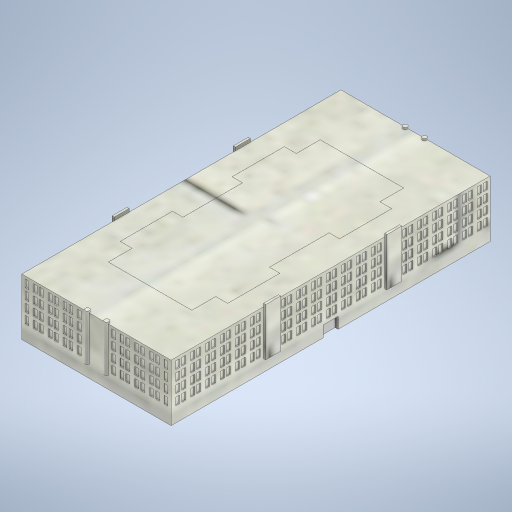
# Autodesk Inventor part: 底部
Saved by Autodesk Inventor 2024.2 (Build 282272000, 272)
## iProperties
Created: 2024-05-15
Part Number: 底部
Material: 一般
Document SubType Name: Modeling
Designer: sohil
Density: 1 g/cm^3
Appearance: 預設
Author: sohil
Autodesk Inventor part; units mm, degrees
(part 1 of 2)
ref_plane "YZ Plane" through (0, 0, 0) normal (1, 0, 0) x (0, 1, 0)
sketch "草圖1" plane through (0, 0, 0) normal (0, 1, 0) x (-1, 0, 0)
  line L0 (20.1844, 27.5664) -> (-79.8156, 27.5664)
  line L1 (-79.8156, 27.5664) -> (-79.8156, -186.2336)
  line L2 (-79.8156, -186.2336) -> (20.1844, -186.2336)
  line L3 (20.1844, -186.2336) -> (20.1844, 27.5664)
  point P0 (0, 0)
  dimension "d0" = 100
  dimension "d1" = 213.8
  constraints: 8 end point, 2 parallel, 1 horizontal, 1 perpendicular
  measures "d0" distance of L2.end L1.end
  measures "d1" distance of L1.end L0.end
extrude "擠出1" add sketch "草圖1" along normal blind 30
sketch "草圖5" plane through (-20.1844, 0, -186.2336) normal (-1, 0, 0) x (0, 0, 1)
  line L0 (1.8826, 27.9757) -> (4.3826, 27.9757)
  line L1 (4.3826, 27.9757) -> (4.3826, 22.9757)
  line L2 (4.3826, 22.9757) -> (1.8826, 22.9757)
  line L3 (1.8826, 22.9757) -> (1.8826, 27.9757)
  line L4 (5.8826, 27.9757) -> (8.3826, 27.9757)
  line L5 (8.3826, 27.9757) -> (8.3826, 22.9757)
  line L6 (8.3826, 22.9757) -> (5.8826, 22.9757)
  line L7 (5.8826, 22.9757) -> (5.8826, 27.9757)
  line L8 (1.8826, 20.9757) -> (4.3826, 20.9757)
  line L9 (4.3826, 20.9757) -> (4.3826, 15.9757)
  line L10 (4.3826, 15.9757) -> (1.8826, 15.9757)
  line L11 (1.8826, 15.9757) -> (1.8826, 20.9757)
  line L12 (5.8826, 20.9757) -> (8.3826, 20.9757)
  line L13 (8.3826, 20.9757) -> (8.3826, 15.9757)
  line L14 (8.3826, 15.9757) -> (5.8826, 15.9757)
  line L15 (5.8826, 15.9757) -> (5.8826, 20.9757)
  line L16 (1.8826, 13.9757) -> (4.3826, 13.9757)
  line L17 (4.3826, 13.9757) -> (4.3826, 8.9757)
  line L18 (4.3826, 8.9757) -> (1.8826, 8.9757)
  line L19 (1.8826, 8.9757) -> (1.8826, 13.9757)
  line L20 (5.8826, 13.9757) -> (8.3826, 13.9757)
  line L21 (8.3826, 13.9757) -> (8.3826, 8.9757)
  line L22 (8.3826, 8.9757) -> (5.8826, 8.9757)
  line L23 (5.8826, 8.9757) -> (5.8826, 13.9757)
  line L24 (1.8826, 6.9757) -> (4.3826, 6.9757)
  line L25 (4.3826, 6.9757) -> (4.3826, 1.9757)
  line L26 (4.3826, 1.9757) -> (1.8826, 1.9757)
  line L27 (1.8826, 1.9757) -> (1.8826, 6.9757)
  line L28 (5.8826, 6.9757) -> (8.3826, 6.9757)
  line L29 (8.3826, 6.9757) -> (8.3826, 1.9757)
  line L30 (8.3826, 1.9757) -> (5.8826, 1.9757)
  line L31 (5.8826, 1.9757) -> (5.8826, 6.9757)
  line L32 (11.8826, 27.9757) -> (14.3826, 27.9757)
  line L33 (11.8826, 22.9757) -> (11.8826, 27.9757)
  line L34 (14.3826, 27.9757) -> (14.3826, 22.9757)
  line L35 (15.8826, 27.9757) -> (18.3826, 27.9757)
  line L36 (15.8826, 22.9757) -> (15.8826, 27.9757)
  line L37 (18.3826, 27.9757) -> (18.3826, 22.9757)
  line L38 (18.3826, 22.9757) -> (15.8826, 22.9757)
  line L39 (14.3826, 22.9757) -> (11.8826, 22.9757)
  line L40 (11.8826, 20.9757) -> (14.3826, 20.9757)
  line L41 (11.8826, 15.9757) -> (11.8826, 20.9757)
  line L42 (14.3826, 20.9757) -> (14.3826, 15.9757)
  line L43 (14.3826, 15.9757) -> (11.8826, 15.9757)
  line L44 (15.8826, 15.9757) -> (15.8826, 20.9757)
  line L45 (15.8826, 20.9757) -> (18.3826, 20.9757)
  line L46 (18.3826, 20.9757) -> (18.3826, 15.9757)
  line L47 (18.3826, 15.9757) -> (15.8826, 15.9757)
  line L48 (11.8826, 13.9757) -> (14.3826, 13.9757)
  line L49 (11.8826, 8.9757) -> (11.8826, 13.9757)
  line L50 (14.3826, 8.9757) -> (11.8826, 8.9757)
  line L51 (14.3826, 13.9757) -> (14.3826, 8.9757)
  line L52 (11.8826, 1.9757) -> (11.8826, 6.9757)
  line L53 (14.3826, 1.9757) -> (11.8826, 1.9757)
  line L54 (14.3826, 6.9757) -> (14.3826, 1.9757)
  line L55 (11.8826, 6.9757) -> (14.3826, 6.9757)
  line L56 (18.3826, 6.9757) -> (18.3826, 1.9757)
  line L57 (15.8826, 6.9757) -> (18.3826, 6.9757)
  line L58 (15.8826, 1.9757) -> (15.8826, 6.9757)
  line L59 (18.3826, 1.9757) -> (15.8826, 1.9757)
  line L60 (15.8826, 8.9757) -> (15.8826, 13.9757)
  line L61 (18.3826, 8.9757) -> (15.8826, 8.9757)
  line L62 (18.3826, 13.9757) -> (18.3826, 8.9757)
  line L63 (15.8826, 13.9757) -> (18.3826, 13.9757)
  line L64 (21.8826, 27.9757) -> (24.3826, 27.9757)
  line L65 (21.8826, 22.9757) -> (21.8826, 27.9757)
  line L66 (24.3826, 27.9757) -> (24.3826, 22.9757)
  line L67 (25.8826, 27.9757) -> (28.3826, 27.9757)
  line L68 (25.8826, 22.9757) -> (25.8826, 27.9757)
  line L69 (28.3826, 27.9757) -> (28.3826, 22.9757)
  line L70 (28.3826, 22.9757) -> (25.8826, 22.9757)
  line L71 (24.3826, 22.9757) -> (21.8826, 22.9757)
  line L72 (21.8826, 20.9757) -> (24.3826, 20.9757)
  line L73 (21.8826, 15.9757) -> (21.8826, 20.9757)
  line L74 (24.3826, 20.9757) -> (24.3826, 15.9757)
  line L75 (24.3826, 15.9757) -> (21.8826, 15.9757)
  line L76 (25.8826, 15.9757) -> (25.8826, 20.9757)
  line L77 (25.8826, 20.9757) -> (28.3826, 20.9757)
  line L78 (28.3826, 20.9757) -> (28.3826, 15.9757)
  line L79 (28.3826, 15.9757) -> (25.8826, 15.9757)
  line L80 (21.8826, 13.9757) -> (24.3826, 13.9757)
  line L81 (21.8826, 8.9757) -> (21.8826, 13.9757)
  line L82 (24.3826, 8.9757) -> (21.8826, 8.9757)
  line L83 (24.3826, 13.9757) -> (24.3826, 8.9757)
  line L84 (21.8826, 1.9757) -> (21.8826, 6.9757)
  line L85 (24.3826, 1.9757) -> (21.8826, 1.9757)
  line L86 (24.3826, 6.9757) -> (24.3826, 1.9757)
  line L87 (21.8826, 6.9757) -> (24.3826, 6.9757)
  line L88 (28.3826, 6.9757) -> (28.3826, 1.9757)
  line L89 (25.8826, 6.9757) -> (28.3826, 6.9757)
  line L90 (25.8826, 1.9757) -> (25.8826, 6.9757)
  line L91 (28.3826, 1.9757) -> (25.8826, 1.9757)
  line L92 (25.8826, 8.9757) -> (25.8826, 13.9757)
  line L93 (28.3826, 8.9757) -> (25.8826, 8.9757)
  line L94 (28.3826, 13.9757) -> (28.3826, 8.9757)
  line L95 (25.8826, 13.9757) -> (28.3826, 13.9757)
  line L96 (31.8826, 27.9757) -> (34.3826, 27.9757)
  line L97 (31.8826, 22.9757) -> (31.8826, 27.9757)
  line L98 (34.3826, 27.9757) -> (34.3826, 22.9757)
  line L99 (35.8826, 27.9757) -> (38.3826, 27.9757)
  line L100 (35.8826, 22.9757) -> (35.8826, 27.9757)
  line L101 (38.3826, 27.9757) -> (38.3826, 22.9757)
  line L102 (38.3826, 22.9757) -> (35.8826, 22.9757)
  line L103 (34.3826, 22.9757) -> (31.8826, 22.9757)
  line L104 (31.8826, 20.9757) -> (34.3826, 20.9757)
  line L105 (31.8826, 15.9757) -> (31.8826, 20.9757)
  line L106 (34.3826, 20.9757) -> (34.3826, 15.9757)
  line L107 (34.3826, 15.9757) -> (31.8826, 15.9757)
  line L108 (35.8826, 15.9757) -> (35.8826, 20.9757)
  line L109 (35.8826, 20.9757) -> (38.3826, 20.9757)
  line L110 (38.3826, 20.9757) -> (38.3826, 15.9757)
  line L111 (38.3826, 15.9757) -> (35.8826, 15.9757)
  line L112 (31.8826, 13.9757) -> (34.3826, 13.9757)
  line L113 (31.8826, 8.9757) -> (31.8826, 13.9757)
  line L114 (34.3826, 8.9757) -> (31.8826, 8.9757)
  line L115 (34.3826, 13.9757) -> (34.3826, 8.9757)
  line L116 (31.8826, 1.9757) -> (31.8826, 6.9757)
  line L117 (34.3826, 1.9757) -> (31.8826, 1.9757)
  line L118 (34.3826, 6.9757) -> (34.3826, 1.9757)
  line L119 (31.8826, 6.9757) -> (34.3826, 6.9757)
  line L120 (38.3826, 6.9757) -> (38.3826, 1.9757)
  line L121 (35.8826, 6.9757) -> (38.3826, 6.9757)
  line L122 (35.8826, 1.9757) -> (35.8826, 6.9757)
  line L123 (38.3826, 1.9757) -> (35.8826, 1.9757)
  line L124 (35.8826, 8.9757) -> (35.8826, 13.9757)
  line L125 (38.3826, 8.9757) -> (35.8826, 8.9757)
  line L126 (38.3826, 13.9757) -> (38.3826, 8.9757)
  line L127 (35.8826, 13.9757) -> (38.3826, 13.9757)
  line L128 (41.8826, 27.9757) -> (44.3826, 27.9757)
  line L129 (41.8826, 22.9757) -> (41.8826, 27.9757)
  line L130 (44.3826, 27.9757) -> (44.3826, 22.9757)
  line L131 (45.8826, 27.9757) -> (48.3826, 27.9757)
  line L132 (45.8826, 22.9757) -> (45.8826, 27.9757)
  line L133 (48.3826, 27.9757) -> (48.3826, 22.9757)
  line L134 (48.3826, 22.9757) -> (45.8826, 22.9757)
  line L135 (44.3826, 22.9757) -> (41.8826, 22.9757)
  line L136 (41.8826, 20.9757) -> (44.3826, 20.9757)
  line L137 (41.8826, 15.9757) -> (41.8826, 20.9757)
  line L138 (44.3826, 20.9757) -> (44.3826, 15.9757)
  line L139 (44.3826, 15.9757) -> (41.8826, 15.9757)
  line L140 (45.8826, 15.9757) -> (45.8826, 20.9757)
  line L141 (45.8826, 20.9757) -> (48.3826, 20.9757)
  line L142 (48.3826, 20.9757) -> (48.3826, 15.9757)
  line L143 (48.3826, 15.9757) -> (45.8826, 15.9757)
  line L144 (41.8826, 13.9757) -> (44.3826, 13.9757)
  line L145 (41.8826, 8.9757) -> (41.8826, 13.9757)
  line L146 (44.3826, 8.9757) -> (41.8826, 8.9757)
  line L147 (44.3826, 13.9757) -> (44.3826, 8.9757)
  line L148 (41.8826, 1.9757) -> (41.8826, 6.9757)
  line L149 (44.3826, 1.9757) -> (41.8826, 1.9757)
  line L150 (44.3826, 6.9757) -> (44.3826, 1.9757)
  line L151 (41.8826, 6.9757) -> (44.3826, 6.9757)
  line L152 (48.3826, 6.9757) -> (48.3826, 1.9757)
  line L153 (45.8826, 6.9757) -> (48.3826, 6.9757)
  line L154 (45.8826, 1.9757) -> (45.8826, 6.9757)
  line L155 (48.3826, 1.9757) -> (45.8826, 1.9757)
  line L156 (45.8826, 8.9757) -> (45.8826, 13.9757)
  line L157 (48.3826, 8.9757) -> (45.8826, 8.9757)
  line L158 (48.3826, 13.9757) -> (48.3826, 8.9757)
  line L159 (45.8826, 13.9757) -> (48.3826, 13.9757)
  line L160 (51.8826, 27.9757) -> (54.3826, 27.9757)
  line L161 (51.8826, 22.9757) -> (51.8826, 27.9757)
  line L162 (54.3826, 27.9757) -> (54.3826, 22.9757)
  line L163 (55.8826, 27.9757) -> (58.3826, 27.9757)
  line L164 (55.8826, 22.9757) -> (55.8826, 27.9757)
  line L165 (58.3826, 27.9757) -> (58.3826, 22.9757)
  line L166 (58.3826, 22.9757) -> (55.8826, 22.9757)
  line L167 (54.3826, 22.9757) -> (51.8826, 22.9757)
  line L168 (51.8826, 20.9757) -> (54.3826, 20.9757)
  line L169 (51.8826, 15.9757) -> (51.8826, 20.9757)
  line L170 (54.3826, 20.9757) -> (54.3826, 15.9757)
  line L171 (54.3826, 15.9757) -> (51.8826, 15.9757)
  line L172 (55.8826, 15.9757) -> (55.8826, 20.9757)
  line L173 (55.8826, 20.9757) -> (58.3826, 20.9757)
  line L174 (58.3826, 20.9757) -> (58.3826, 15.9757)
  line L175 (58.3826, 15.9757) -> (55.8826, 15.9757)
  line L176 (51.8826, 13.9757) -> (54.3826, 13.9757)
  line L177 (51.8826, 8.9757) -> (51.8826, 13.9757)
  line L178 (54.3826, 8.9757) -> (51.8826, 8.9757)
  line L179 (54.3826, 13.9757) -> (54.3826, 8.9757)
  line L180 (51.8826, 1.9757) -> (51.8826, 6.9757)
  line L181 (54.3826, 1.9757) -> (51.8826, 1.9757)
  line L182 (54.3826, 6.9757) -> (54.3826, 1.9757)
  line L183 (51.8826, 6.9757) -> (54.3826, 6.9757)
  line L184 (58.3826, 6.9757) -> (58.3826, 1.9757)
  line L185 (55.8826, 6.9757) -> (58.3826, 6.9757)
  line L186 (55.8826, 1.9757) -> (55.8826, 6.9757)
  line L187 (58.3826, 1.9757) -> (55.8826, 1.9757)
  line L188 (55.8826, 8.9757) -> (55.8826, 13.9757)
  line L189 (58.3826, 8.9757) -> (55.8826, 8.9757)
  line L190 (58.3826, 13.9757) -> (58.3826, 8.9757)
  line L191 (55.8826, 13.9757) -> (58.3826, 13.9757)
  line L192 (213.8, 0) -> (0, 0) projected
  line L193 (60.6612, 32.0439) -> (70.6612, 32.0439)
  line L194 (70.6612, 32.0439) -> (70.6612, 0)
  line L195 (70.6612, 0) -> (60.6612, 0)
  line L196 (60.6612, 0) -> (60.6612, 32.0439)
  line L197 (73.0512, 27.9757) -> (75.5512, 27.9757)
  line L198 (75.5512, 27.9757) -> (75.5512, 22.9757)
  line L199 (75.5512, 22.9757) -> (73.0512, 22.9757)
  line L200 (73.0512, 22.9757) -> (73.0512, 27.9757)
  line L201 (77.0512, 27.9757) -> (79.5512, 27.9757)
  line L202 (77.0512, 22.9757) -> (77.0512, 27.9757)
  line L203 (79.5512, 27.9757) -> (79.5512, 22.9757)
  line L204 (79.5512, 22.9757) -> (77.0512, 22.9757)
  line L205 (73.0512, 20.9757) -> (75.5512, 20.9757)
  line L206 (73.0512, 15.9757) -> (73.0512, 20.9757)
  line L207 (75.5512, 20.9757) -> (75.5512, 15.9757)
  line L208 (75.5512, 15.9757) -> (73.0512, 15.9757)
  line L209 (77.0512, 20.9757) -> (79.5512, 20.9757)
  line L210 (77.0512, 15.9757) -> (77.0512, 20.9757)
  line L211 (79.5512, 20.9757) -> (79.5512, 15.9757)
  line L212 (79.5512, 15.9757) -> (77.0512, 15.9757)
  line L213 (73.0512, 13.9757) -> (75.5512, 13.9757)
  line L214 (73.0512, 8.9757) -> (73.0512, 13.9757)
  line L215 (75.5512, 13.9757) -> (75.5512, 8.9757)
  line L216 (75.5512, 8.9757) -> (73.0512, 8.9757)
  line L217 (77.0512, 13.9757) -> (79.5512, 13.9757)
  line L218 (77.0512, 8.9757) -> (77.0512, 13.9757)
  line L219 (79.5512, 13.9757) -> (79.5512, 8.9757)
  line L220 (79.5512, 8.9757) -> (77.0512, 8.9757)
  line L221 (73.0512, 6.9757) -> (75.5512, 6.9757)
  line L222 (73.0512, 1.9757) -> (73.0512, 6.9757)
  line L223 (75.5512, 6.9757) -> (75.5512, 1.9757)
  line L224 (75.5512, 1.9757) -> (73.0512, 1.9757)
  line L225 (77.0512, 6.9757) -> (79.5512, 6.9757)
  line L226 (77.0512, 1.9757) -> (77.0512, 6.9757)
  line L227 (79.5512, 6.9757) -> (79.5512, 1.9757)
  line L228 (79.5512, 1.9757) -> (77.0512, 1.9757)
  line L229 (89.5512, 22.9757) -> (87.0512, 22.9757)
  line L230 (85.5512, 22.9757) -> (83.0512, 22.9757)
  line L231 (83.0512, 22.9757) -> (83.0512, 27.9757)
  line L232 (83.0512, 27.9757) -> (85.5512, 27.9757)
  line L233 (85.5512, 27.9757) -> (85.5512, 22.9757)
  line L234 (87.0512, 27.9757) -> (89.5512, 27.9757)
  line L235 (89.5512, 27.9757) -> (89.5512, 22.9757)
  line L236 (87.0512, 22.9757) -> (87.0512, 27.9757)
  line L237 (83.0512, 13.9757) -> (85.5512, 13.9757)
  line L238 (87.0512, 13.9757) -> (89.5512, 13.9757)
  line L239 (89.5512, 8.9757) -> (87.0512, 8.9757)
  line L240 (89.5512, 13.9757) -> (89.5512, 8.9757)
  line L241 (87.0512, 8.9757) -> (87.0512, 13.9757)
  line L242 (85.5512, 13.9757) -> (85.5512, 8.9757)
  line L243 (85.5512, 8.9757) -> (83.0512, 8.9757)
  line L244 (83.0512, 8.9757) -> (83.0512, 13.9757)
  line L245 (83.0512, 6.9757) -> (85.5512, 6.9757)
  line L246 (87.0512, 6.9757) -> (89.5512, 6.9757)
  line L247 (89.5512, 6.9757) -> (89.5512, 1.9757)
  line L248 (89.5512, 1.9757) -> (87.0512, 1.9757)
  line L249 (83.0512, 1.9757) -> (83.0512, 6.9757)
  line L250 (85.5512, 6.9757) -> (85.5512, 1.9757)
  line L251 (87.0512, 1.9757) -> (87.0512, 6.9757)
  line L252 (85.5512, 1.9757) -> (83.0512, 1.9757)
  line L253 (83.0512, 20.9757) -> (85.5512, 20.9757)
  line L254 (87.0512, 20.9757) -> (89.5512, 20.9757)
  line L255 (89.5512, 15.9757) -> (87.0512, 15.9757)
  line L256 (89.5512, 20.9757) -> (89.5512, 15.9757)
  line L257 (87.0512, 15.9757) -> (87.0512, 20.9757)
  line L258 (85.5512, 20.9757) -> (85.5512, 15.9757)
  line L259 (83.0512, 15.9757) -> (83.0512, 20.9757)
  line L260 (85.5512, 15.9757) -> (83.0512, 15.9757)
  line L261 (99.5512, 22.9757) -> (97.0512, 22.9757)
  line L262 (95.5512, 22.9757) -> (93.0512, 22.9757)
  line L263 (93.0512, 22.9757) -> (93.0512, 27.9757)
  line L264 (93.0512, 27.9757) -> (95.5512, 27.9757)
  line L265 (95.5512, 27.9757) -> (95.5512, 22.9757)
  line L266 (97.0512, 27.9757) -> (99.5512, 27.9757)
  line L267 (99.5512, 27.9757) -> (99.5512, 22.9757)
  line L268 (97.0512, 22.9757) -> (97.0512, 27.9757)
  line L269 (93.0512, 13.9757) -> (95.5512, 13.9757)
  line L270 (97.0512, 13.9757) -> (99.5512, 13.9757)
  line L271 (99.5512, 8.9757) -> (97.0512, 8.9757)
  line L272 (99.5512, 13.9757) -> (99.5512, 8.9757)
  line L273 (97.0512, 8.9757) -> (97.0512, 13.9757)
  line L274 (95.5512, 13.9757) -> (95.5512, 8.9757)
  line L275 (95.5512, 8.9757) -> (93.0512, 8.9757)
  line L276 (93.0512, 8.9757) -> (93.0512, 13.9757)
  line L277 (93.0512, 6.9757) -> (95.5512, 6.9757)
  line L278 (97.0512, 6.9757) -> (99.5512, 6.9757)
  line L279 (99.5512, 6.9757) -> (99.5512, 1.9757)
  line L280 (99.5512, 1.9757) -> (97.0512, 1.9757)
  line L281 (93.0512, 1.9757) -> (93.0512, 6.9757)
  line L282 (95.5512, 6.9757) -> (95.5512, 1.9757)
  line L283 (97.0512, 1.9757) -> (97.0512, 6.9757)
  line L284 (95.5512, 1.9757) -> (93.0512, 1.9757)
  line L285 (93.0512, 20.9757) -> (95.5512, 20.9757)
  line L286 (97.0512, 20.9757) -> (99.5512, 20.9757)
  line L287 (99.5512, 15.9757) -> (97.0512, 15.9757)
  line L288 (99.5512, 20.9757) -> (99.5512, 15.9757)
  line L289 (97.0512, 15.9757) -> (97.0512, 20.9757)
  line L290 (95.5512, 20.9757) -> (95.5512, 15.9757)
  line L291 (93.0512, 15.9757) -> (93.0512, 20.9757)
  line L292 (95.5512, 15.9757) -> (93.0512, 15.9757)
  line L293 (109.5512, 22.9757) -> (107.0512, 22.9757)
  line L294 (105.5512, 22.9757) -> (103.0512, 22.9757)
  line L295 (103.0512, 22.9757) -> (103.0512, 27.9757)
  line L296 (103.0512, 27.9757) -> (105.5512, 27.9757)
  line L297 (105.5512, 27.9757) -> (105.5512, 22.9757)
  line L298 (107.0512, 27.9757) -> (109.5512, 27.9757)
  line L299 (109.5512, 27.9757) -> (109.5512, 22.9757)
  line L300 (107.0512, 22.9757) -> (107.0512, 27.9757)
  line L301 (103.0512, 13.9757) -> (105.5512, 13.9757)
  line L302 (107.0512, 13.9757) -> (109.5512, 13.9757)
  line L303 (109.5512, 8.9757) -> (107.0512, 8.9757)
  line L304 (109.5512, 13.9757) -> (109.5512, 8.9757)
  line L305 (107.0512, 8.9757) -> (107.0512, 13.9757)
  line L306 (105.5512, 13.9757) -> (105.5512, 8.9757)
  line L307 (105.5512, 8.9757) -> (103.0512, 8.9757)
  line L308 (103.0512, 8.9757) -> (103.0512, 13.9757)
  line L309 (103.0512, 6.9757) -> (105.5512, 6.9757)
  line L310 (107.0512, 6.9757) -> (109.5512, 6.9757)
  line L311 (109.5512, 6.9757) -> (109.5512, 1.9757)
  line L312 (109.5512, 1.9757) -> (107.0512, 1.9757)
  line L313 (103.0512, 1.9757) -> (103.0512, 6.9757)
  line L314 (105.5512, 6.9757) -> (105.5512, 1.9757)
  line L315 (107.0512, 1.9757) -> (107.0512, 6.9757)
  line L316 (105.5512, 1.9757) -> (103.0512, 1.9757)
  line L317 (103.0512, 20.9757) -> (105.5512, 20.9757)
  line L318 (107.0512, 20.9757) -> (109.5512, 20.9757)
  line L319 (109.5512, 15.9757) -> (107.0512, 15.9757)
  line L320 (109.5512, 20.9757) -> (109.5512, 15.9757)
  line L321 (107.0512, 15.9757) -> (107.0512, 20.9757)
  line L322 (105.5512, 20.9757) -> (105.5512, 15.9757)
  line L323 (103.0512, 15.9757) -> (103.0512, 20.9757)
  line L324 (105.5512, 15.9757) -> (103.0512, 15.9757)
  line L325 (119.5512, 22.9757) -> (117.0512, 22.9757)
  line L326 (115.5512, 22.9757) -> (113.0512, 22.9757)
  line L327 (113.0512, 22.9757) -> (113.0512, 27.9757)
  line L328 (113.0512, 27.9757) -> (115.5512, 27.9757)
  line L329 (115.5512, 27.9757) -> (115.5512, 22.9757)
  line L330 (117.0512, 27.9757) -> (119.5512, 27.9757)
  line L331 (119.5512, 27.9757) -> (119.5512, 22.9757)
  line L332 (117.0512, 22.9757) -> (117.0512, 27.9757)
  line L333 (113.0512, 13.9757) -> (115.5512, 13.9757)
  line L334 (117.0512, 13.9757) -> (119.5512, 13.9757)
  line L335 (119.5512, 8.9757) -> (117.0512, 8.9757)
  line L336 (119.5512, 13.9757) -> (119.5512, 8.9757)
  line L337 (117.0512, 8.9757) -> (117.0512, 13.9757)
  line L338 (115.5512, 13.9757) -> (115.5512, 8.9757)
  line L339 (115.5512, 8.9757) -> (113.0512, 8.9757)
  line L340 (113.0512, 8.9757) -> (113.0512, 13.9757)
  line L341 (113.0512, 6.9757) -> (115.5512, 6.9757)
  line L342 (117.0512, 6.9757) -> (119.5512, 6.9757)
  line L343 (119.5512, 6.9757) -> (119.5512, 1.9757)
  line L344 (119.5512, 1.9757) -> (117.0512, 1.9757)
  line L345 (113.0512, 1.9757) -> (113.0512, 6.9757)
  line L346 (115.5512, 6.9757) -> (115.5512, 1.9757)
  line L347 (117.0512, 1.9757) -> (117.0512, 6.9757)
  line L348 (115.5512, 1.9757) -> (113.0512, 1.9757)
  line L349 (113.0512, 20.9757) -> (115.5512, 20.9757)
  line L350 (117.0512, 20.9757) -> (119.5512, 20.9757)
  line L351 (119.5512, 15.9757) -> (117.0512, 15.9757)
  line L352 (119.5512, 20.9757) -> (119.5512, 15.9757)
  line L353 (117.0512, 15.9757) -> (117.0512, 20.9757)
  line L354 (115.5512, 20.9757) -> (115.5512, 15.9757)
  line L355 (113.0512, 15.9757) -> (113.0512, 20.9757)
  line L356 (115.5512, 15.9757) -> (113.0512, 15.9757)
  line L357 (129.5512, 22.9757) -> (127.0512, 22.9757)
  line L358 (125.5512, 22.9757) -> (123.0512, 22.9757)
  line L359 (123.0512, 22.9757) -> (123.0512, 27.9757)
  line L360 (123.0512, 27.9757) -> (125.5512, 27.9757)
  line L361 (125.5512, 27.9757) -> (125.5512, 22.9757)
  line L362 (127.0512, 27.9757) -> (129.5512, 27.9757)
  line L363 (129.5512, 27.9757) -> (129.5512, 22.9757)
  line L364 (127.0512, 22.9757) -> (127.0512, 27.9757)
  line L365 (123.0512, 13.9757) -> (125.5512, 13.9757)
  line L366 (127.0512, 13.9757) -> (129.5512, 13.9757)
  line L367 (129.5512, 8.9757) -> (127.0512, 8.9757)
  line L368 (129.5512, 13.9757) -> (129.5512, 8.9757)
  line L369 (127.0512, 8.9757) -> (127.0512, 13.9757)
  line L370 (125.5512, 13.9757) -> (125.5512, 8.9757)
  line L371 (125.5512, 8.9757) -> (123.0512, 8.9757)
  line L372 (123.0512, 8.9757) -> (123.0512, 13.9757)
  line L373 (123.0512, 6.9757) -> (125.5512, 6.9757)
  line L374 (127.0512, 6.9757) -> (129.5512, 6.9757)
  line L375 (129.5512, 6.9757) -> (129.5512, 1.9757)
  line L376 (129.5512, 1.9757) -> (127.0512, 1.9757)
  line L377 (123.0512, 1.9757) -> (123.0512, 6.9757)
  line L378 (125.5512, 6.9757) -> (125.5512, 1.9757)
  line L379 (127.0512, 1.9757) -> (127.0512, 6.9757)
  line L380 (125.5512, 1.9757) -> (123.0512, 1.9757)
  line L381 (123.0512, 20.9757) -> (125.5512, 20.9757)
  line L382 (127.0512, 20.9757) -> (129.5512, 20.9757)
  line L383 (129.5512, 15.9757) -> (127.0512, 15.9757)
  line L384 (129.5512, 20.9757) -> (129.5512, 15.9757)
  line L385 (127.0512, 15.9757) -> (127.0512, 20.9757)
  line L386 (125.5512, 20.9757) -> (125.5512, 15.9757)
  line L387 (123.0512, 15.9757) -> (123.0512, 20.9757)
  line L388 (125.5512, 15.9757) -> (123.0512, 15.9757)
  line L389 (139.5512, 22.9757) -> (137.0512, 22.9757)
  line L390 (135.5512, 22.9757) -> (133.0512, 22.9757)
  line L391 (133.0512, 22.9757) -> (133.0512, 27.9757)
  line L392 (133.0512, 27.9757) -> (135.5512, 27.9757)
  line L393 (135.5512, 27.9757) -> (135.5512, 22.9757)
  line L394 (137.0512, 27.9757) -> (139.5512, 27.9757)
  line L395 (139.5512, 27.9757) -> (139.5512, 22.9757)
  line L396 (137.0512, 22.9757) -> (137.0512, 27.9757)
  line L397 (133.0512, 13.9757) -> (135.5512, 13.9757)
  line L398 (137.0512, 13.9757) -> (139.5512, 13.9757)
  line L399 (139.5512, 8.9757) -> (137.0512, 8.9757)
  line L400 (139.5512, 13.9757) -> (139.5512, 8.9757)
  line L401 (137.0512, 8.9757) -> (137.0512, 13.9757)
  line L402 (135.5512, 13.9757) -> (135.5512, 8.9757)
  line L403 (135.5512, 8.9757) -> (133.0512, 8.9757)
  line L404 (133.0512, 8.9757) -> (133.0512, 13.9757)
  line L405 (133.0512, 6.9757) -> (135.5512, 6.9757)
  line L406 (137.0512, 6.9757) -> (139.5512, 6.9757)
  line L407 (139.5512, 6.9757) -> (139.5512, 1.9757)
  line L408 (139.5512, 1.9757) -> (137.0512, 1.9757)
  line L409 (133.0512, 1.9757) -> (133.0512, 6.9757)
  line L410 (135.5512, 6.9757) -> (135.5512, 1.9757)
  line L411 (137.0512, 1.9757) -> (137.0512, 6.9757)
  line L412 (135.5512, 1.9757) -> (133.0512, 1.9757)
  line L413 (133.0512, 20.9757) -> (135.5512, 20.9757)
  line L414 (137.0512, 20.9757) -> (139.5512, 20.9757)
  line L415 (139.5512, 15.9757) -> (137.0512, 15.9757)
  line L416 (139.5512, 20.9757) -> (139.5512, 15.9757)
  line L417 (137.0512, 15.9757) -> (137.0512, 20.9757)
  line L418 (135.5512, 20.9757) -> (135.5512, 15.9757)
  line L419 (133.0512, 15.9757) -> (133.0512, 20.9757)
  line L420 (135.5512, 15.9757) -> (133.0512, 15.9757)
  line L421 (141.8302, 32.0439) -> (151.8302, 32.0439)
  line L422 (151.8302, 32.0439) -> (151.8302, 0)
  line L423 (151.8302, 0) -> (141.8302, 0)
  line L424 (141.8302, 0) -> (141.8302, 32.0439)
  line L425 (154.1092, 27.9757) -> (156.6092, 27.9757)
  line L426 (156.6092, 27.9757) -> (156.6092, 22.9757)
  line L427 (156.6092, 22.9757) -> (154.1092, 22.9757)
  line L428 (154.1092, 22.9757) -> (154.1092, 27.9757)
  line L429 (160.6092, 22.9757) -> (158.1092, 22.9757)
  line L430 (158.1092, 22.9757) -> (158.1092, 27.9757)
  line L431 (158.1092, 27.9757) -> (160.6092, 27.9757)
  line L432 (160.6092, 27.9757) -> (160.6092, 22.9757)
  line L433 (156.6092, 15.9757) -> (154.1092, 15.9757)
  line L434 (154.1092, 15.9757) -> (154.1092, 20.9757)
  line L435 (154.1092, 20.9757) -> (156.6092, 20.9757)
  line L436 (156.6092, 20.9757) -> (156.6092, 15.9757)
  line L437 (160.6092, 15.9757) -> (158.1092, 15.9757)
  line L438 (158.1092, 15.9757) -> (158.1092, 20.9757)
  line L439 (158.1092, 20.9757) -> (160.6092, 20.9757)
  line L440 (160.6092, 20.9757) -> (160.6092, 15.9757)
  line L441 (156.6092, 8.9757) -> (154.1092, 8.9757)
  line L442 (154.1092, 8.9757) -> (154.1092, 13.9757)
  line L443 (154.1092, 13.9757) -> (156.6092, 13.9757)
  line L444 (156.6092, 13.9757) -> (156.6092, 8.9757)
  line L445 (160.6092, 8.9757) -> (158.1092, 8.9757)
  line L446 (158.1092, 8.9757) -> (158.1092, 13.9757)
  line L447 (158.1092, 13.9757) -> (160.6092, 13.9757)
  line L448 (160.6092, 13.9757) -> (160.6092, 8.9757)
  line L449 (156.6092, 1.9757) -> (154.1092, 1.9757)
  line L450 (154.1092, 1.9757) -> (154.1092, 6.9757)
  line L451 (154.1092, 6.9757) -> (156.6092, 6.9757)
  line L452 (156.6092, 6.9757) -> (156.6092, 1.9757)
  line L453 (160.6092, 1.9757) -> (158.1092, 1.9757)
  line L454 (158.1092, 1.9757) -> (158.1092, 6.9757)
  line L455 (158.1092, 6.9757) -> (160.6092, 6.9757)
  line L456 (160.6092, 6.9757) -> (160.6092, 1.9757)
  line L457 (168.1092, 20.9757) -> (170.6092, 20.9757)
  line L458 (164.1092, 20.9757) -> (166.6092, 20.9757)
  line L459 (166.6092, 15.9757) -> (164.1092, 15.9757)
  line L460 (164.1092, 15.9757) -> (164.1092, 20.9757)
  line L461 (166.6092, 20.9757) -> (166.6092, 15.9757)
  line L462 (168.1092, 15.9757) -> (168.1092, 20.9757)
  line L463 (170.6092, 20.9757) -> (170.6092, 15.9757)
  line L464 (170.6092, 15.9757) -> (168.1092, 15.9757)
  line L465 (168.1092, 13.9757) -> (170.6092, 13.9757)
  line L466 (164.1092, 13.9757) -> (166.6092, 13.9757)
  line L467 (164.1092, 8.9757) -> (164.1092, 13.9757)
  line L468 (166.6092, 8.9757) -> (164.1092, 8.9757)
  line L469 (166.6092, 13.9757) -> (166.6092, 8.9757)
  line L470 (168.1092, 8.9757) -> (168.1092, 13.9757)
  line L471 (170.6092, 13.9757) -> (170.6092, 8.9757)
  line L472 (170.6092, 8.9757) -> (168.1092, 8.9757)
  line L473 (164.1092, 22.9757) -> (164.1092, 27.9757)
  line L474 (166.6092, 22.9757) -> (164.1092, 22.9757)
  line L475 (164.1092, 27.9757) -> (166.6092, 27.9757)
  line L476 (166.6092, 27.9757) -> (166.6092, 22.9757)
  line L477 (168.1092, 22.9757) -> (168.1092, 27.9757)
  line L478 (170.6092, 22.9757) -> (168.1092, 22.9757)
  line L479 (168.1092, 27.9757) -> (170.6092, 27.9757)
  line L480 (170.6092, 27.9757) -> (170.6092, 22.9757)
  line L481 (164.1092, 6.9757) -> (166.6092, 6.9757)
  line L482 (168.1092, 6.9757) -> (170.6092, 6.9757)
  line L483 (166.6092, 1.9757) -> (164.1092, 1.9757)
  line L484 (164.1092, 1.9757) -> (164.1092, 6.9757)
  line L485 (166.6092, 6.9757) -> (166.6092, 1.9757)
  line L486 (168.1092, 1.9757) -> (168.1092, 6.9757)
  line L487 (170.6092, 6.9757) -> (170.6092, 1.9757)
  line L488 (170.6092, 1.9757) -> (168.1092, 1.9757)
  line L489 (178.1092, 20.9757) -> (180.6092, 20.9757)
  line L490 (174.1092, 20.9757) -> (176.6092, 20.9757)
  line L491 (176.6092, 15.9757) -> (174.1092, 15.9757)
  line L492 (174.1092, 15.9757) -> (174.1092, 20.9757)
  line L493 (176.6092, 20.9757) -> (176.6092, 15.9757)
  line L494 (178.1092, 15.9757) -> (178.1092, 20.9757)
  line L495 (180.6092, 20.9757) -> (180.6092, 15.9757)
  line L496 (180.6092, 15.9757) -> (178.1092, 15.9757)
  line L497 (178.1092, 13.9757) -> (180.6092, 13.9757)
  line L498 (174.1092, 13.9757) -> (176.6092, 13.9757)
  line L499 (174.1092, 8.9757) -> (174.1092, 13.9757)
  line L500 (176.6092, 8.9757) -> (174.1092, 8.9757)
  line L501 (176.6092, 13.9757) -> (176.6092, 8.9757)
  line L502 (178.1092, 8.9757) -> (178.1092, 13.9757)
  line L503 (180.6092, 13.9757) -> (180.6092, 8.9757)
  line L504 (180.6092, 8.9757) -> (178.1092, 8.9757)
  line L505 (174.1092, 22.9757) -> (174.1092, 27.9757)
  line L506 (176.6092, 22.9757) -> (174.1092, 22.9757)
  line L507 (174.1092, 27.9757) -> (176.6092, 27.9757)
  line L508 (176.6092, 27.9757) -> (176.6092, 22.9757)
  line L509 (178.1092, 22.9757) -> (178.1092, 27.9757)
  line L510 (180.6092, 22.9757) -> (178.1092, 22.9757)
  line L511 (178.1092, 27.9757) -> (180.6092, 27.9757)
  line L512 (180.6092, 27.9757) -> (180.6092, 22.9757)
  line L513 (174.1092, 6.9757) -> (176.6092, 6.9757)
  line L514 (178.1092, 6.9757) -> (180.6092, 6.9757)
  line L515 (176.6092, 1.9757) -> (174.1092, 1.9757)
  line L516 (174.1092, 1.9757) -> (174.1092, 6.9757)
  line L517 (176.6092, 6.9757) -> (176.6092, 1.9757)
  line L518 (178.1092, 1.9757) -> (178.1092, 6.9757)
  line L519 (180.6092, 6.9757) -> (180.6092, 1.9757)
  line L520 (180.6092, 1.9757) -> (178.1092, 1.9757)
  line L521 (188.1092, 20.9757) -> (190.6092, 20.9757)
  line L522 (184.1092, 20.9757) -> (186.6092, 20.9757)
  line L523 (186.6092, 15.9757) -> (184.1092, 15.9757)
  line L524 (184.1092, 15.9757) -> (184.1092, 20.9757)
  line L525 (186.6092, 20.9757) -> (186.6092, 15.9757)
  line L526 (188.1092, 15.9757) -> (188.1092, 20.9757)
  line L527 (190.6092, 20.9757) -> (190.6092, 15.9757)
  line L528 (190.6092, 15.9757) -> (188.1092, 15.9757)
  line L529 (188.1092, 13.9757) -> (190.6092, 13.9757)
  line L530 (184.1092, 13.9757) -> (186.6092, 13.9757)
  line L531 (184.1092, 8.9757) -> (184.1092, 13.9757)
  line L532 (186.6092, 8.9757) -> (184.1092, 8.9757)
  line L533 (186.6092, 13.9757) -> (186.6092, 8.9757)
  line L534 (188.1092, 8.9757) -> (188.1092, 13.9757)
  line L535 (190.6092, 13.9757) -> (190.6092, 8.9757)
  line L536 (190.6092, 8.9757) -> (188.1092, 8.9757)
  line L537 (184.1092, 22.9757) -> (184.1092, 27.9757)
  line L538 (186.6092, 22.9757) -> (184.1092, 22.9757)
  line L539 (184.1092, 27.9757) -> (186.6092, 27.9757)
  line L540 (186.6092, 27.9757) -> (186.6092, 22.9757)
  line L541 (188.1092, 22.9757) -> (188.1092, 27.9757)
  line L542 (190.6092, 22.9757) -> (188.1092, 22.9757)
  line L543 (188.1092, 27.9757) -> (190.6092, 27.9757)
  line L544 (190.6092, 27.9757) -> (190.6092, 22.9757)
  line L545 (184.1092, 6.9757) -> (186.6092, 6.9757)
  line L546 (188.1092, 6.9757) -> (190.6092, 6.9757)
  line L547 (186.6092, 1.9757) -> (184.1092, 1.9757)
  line L548 (184.1092, 1.9757) -> (184.1092, 6.9757)
  line L549 (186.6092, 6.9757) -> (186.6092, 1.9757)
  line L550 (188.1092, 1.9757) -> (188.1092, 6.9757)
  line L551 (190.6092, 6.9757) -> (190.6092, 1.9757)
  line L552 (190.6092, 1.9757) -> (188.1092, 1.9757)
  line L553 (198.1092, 20.9757) -> (200.6092, 20.9757)
  line L554 (194.1092, 20.9757) -> (196.6092, 20.9757)
  line L555 (196.6092, 15.9757) -> (194.1092, 15.9757)
  line L556 (194.1092, 15.9757) -> (194.1092, 20.9757)
  line L557 (196.6092, 20.9757) -> (196.6092, 15.9757)
  line L558 (198.1092, 15.9757) -> (198.1092, 20.9757)
  line L559 (200.6092, 20.9757) -> (200.6092, 15.9757)
  line L560 (200.6092, 15.9757) -> (198.1092, 15.9757)
  line L561 (198.1092, 13.9757) -> (200.6092, 13.9757)
  line L562 (194.1092, 13.9757) -> (196.6092, 13.9757)
  line L563 (194.1092, 8.9757) -> (194.1092, 13.9757)
  line L564 (196.6092, 8.9757) -> (194.1092, 8.9757)
  line L565 (196.6092, 13.9757) -> (196.6092, 8.9757)
  line L566 (198.1092, 8.9757) -> (198.1092, 13.9757)
  line L567 (200.6092, 13.9757) -> (200.6092, 8.9757)
  line L568 (200.6092, 8.9757) -> (198.1092, 8.9757)
  line L569 (194.1092, 22.9757) -> (194.1092, 27.9757)
  line L570 (196.6092, 22.9757) -> (194.1092, 22.9757)
  line L571 (194.1092, 27.9757) -> (196.6092, 27.9757)
  line L572 (196.6092, 27.9757) -> (196.6092, 22.9757)
  line L573 (198.1092, 22.9757) -> (198.1092, 27.9757)
  line L574 (200.6092, 22.9757) -> (198.1092, 22.9757)
  line L575 (198.1092, 27.9757) -> (200.6092, 27.9757)
  line L576 (200.6092, 27.9757) -> (200.6092, 22.9757)
  line L577 (194.1092, 6.9757) -> (196.6092, 6.9757)
  line L578 (198.1092, 6.9757) -> (200.6092, 6.9757)
  line L579 (196.6092, 1.9757) -> (194.1092, 1.9757)
  line L580 (194.1092, 1.9757) -> (194.1092, 6.9757)
  line L581 (196.6092, 6.9757) -> (196.6092, 1.9757)
  line L582 (198.1092, 1.9757) -> (198.1092, 6.9757)
  line L583 (200.6092, 6.9757) -> (200.6092, 1.9757)
  line L584 (200.6092, 1.9757) -> (198.1092, 1.9757)
  line L585 (208.1092, 20.9757) -> (210.6092, 20.9757)
  line L586 (204.1092, 20.9757) -> (206.6092, 20.9757)
  line L587 (206.6092, 15.9757) -> (204.1092, 15.9757)
  line L588 (204.1092, 15.9757) -> (204.1092, 20.9757)
  line L589 (206.6092, 20.9757) -> (206.6092, 15.9757)
  line L590 (208.1092, 15.9757) -> (208.1092, 20.9757)
  line L591 (210.6092, 20.9757) -> (210.6092, 15.9757)
  line L592 (210.6092, 15.9757) -> (208.1092, 15.9757)
  line L593 (208.1092, 13.9757) -> (210.6092, 13.9757)
  line L594 (204.1092, 13.9757) -> (206.6092, 13.9757)
  line L595 (204.1092, 8.9757) -> (204.1092, 13.9757)
  line L596 (206.6092, 8.9757) -> (204.1092, 8.9757)
  line L597 (206.6092, 13.9757) -> (206.6092, 8.9757)
  line L598 (208.1092, 8.9757) -> (208.1092, 13.9757)
  line L599 (210.6092, 13.9757) -> (210.6092, 8.9757)
  line L600 (210.6092, 8.9757) -> (208.1092, 8.9757)
  line L601 (204.1092, 22.9757) -> (204.1092, 27.9757)
  line L602 (206.6092, 22.9757) -> (204.1092, 22.9757)
  line L603 (204.1092, 27.9757) -> (206.6092, 27.9757)
  line L604 (206.6092, 27.9757) -> (206.6092, 22.9757)
  line L605 (208.1092, 22.9757) -> (208.1092, 27.9757)
  line L606 (210.6092, 22.9757) -> (208.1092, 22.9757)
  line L607 (208.1092, 27.9757) -> (210.6092, 27.9757)
  line L608 (210.6092, 27.9757) -> (210.6092, 22.9757)
  line L609 (204.1092, 6.9757) -> (206.6092, 6.9757)
  line L610 (208.1092, 6.9757) -> (210.6092, 6.9757)
  line L611 (206.6092, 1.9757) -> (204.1092, 1.9757)
  line L612 (204.1092, 1.9757) -> (204.1092, 6.9757)
  line L613 (206.6092, 6.9757) -> (206.6092, 1.9757)
  line L614 (208.1092, 1.9757) -> (208.1092, 6.9757)
  line L615 (210.6092, 6.9757) -> (210.6092, 1.9757)
  line L616 (210.6092, 1.9757) -> (208.1092, 1.9757)
  point P0 (186.2336, 0)
  point P1 (154.1092, 25.4757)
  point P2 (158.1092, 25.4757)
  point P3 (154.1092, 18.4757)
  point P4 (158.1092, 18.4757)
  point P5 (154.1092, 11.4757)
  point P6 (158.1092, 11.4757)
  point P7 (154.1092, 4.4757)
  point P8 (158.1092, 4.4757)
  point P9 (164.1092, 18.4757)
  point P10 (168.1092, 18.4757)
  point P11 (164.1092, 11.4757)
  point P12 (168.1092, 11.4757)
  point P13 (164.1092, 25.4757)
  point P14 (168.1092, 25.4757)
  point P15 (164.1092, 4.4757)
  point P16 (168.1092, 4.4757)
  point P17 (174.1092, 18.4757)
  point P18 (178.1092, 18.4757)
  point P19 (174.1092, 11.4757)
  point P20 (178.1092, 11.4757)
  point P21 (174.1092, 25.4757)
  point P22 (178.1092, 25.4757)
  point P23 (174.1092, 4.4757)
  point P24 (178.1092, 4.4757)
  point P25 (184.1092, 18.4757)
  point P26 (188.1092, 18.4757)
  point P27 (184.1092, 11.4757)
  point P28 (188.1092, 11.4757)
  point P29 (184.1092, 25.4757)
  point P30 (188.1092, 25.4757)
  point P31 (184.1092, 4.4757)
  point P32 (188.1092, 4.4757)
  point P33 (194.1092, 18.4757)
  point P34 (198.1092, 18.4757)
  point P35 (194.1092, 11.4757)
  point P36 (198.1092, 11.4757)
  point P37 (194.1092, 25.4757)
  point P38 (198.1092, 25.4757)
  point P39 (194.1092, 4.4757)
  point P40 (198.1092, 4.4757)
  point P41 (204.1092, 18.4757)
  point P42 (208.1092, 18.4757)
  point P43 (204.1092, 11.4757)
  point P44 (208.1092, 11.4757)
  point P45 (204.1092, 25.4757)
  point P46 (208.1092, 25.4757)
  point P47 (204.1092, 4.4757)
  point P48 (208.1092, 4.4757)
  dimension "d164" = 2.5
  dimension "d165" = 5
  dimension "d168" = 4
  dimension "d171" = 7
  dimension "d176" = 10
  dimension "d181" = 10
  dimension "d189" = 2.5
  dimension "d190" = 5
  dimension "d193" = 4
  dimension "d196" = 7
  dimension "d201" = 10
  dimension "d206" = 10
  dimension "d207" = 2.5
  dimension "d208" = 2.279
  dimension "d209" = 2.279
  dimension "d212" = 4
  dimension "d215" = 7
  dimension "d220" = 10
  dimension "d225" = 2.2786
  constraints: 1232 end point, 11 horizontal, 10 parallel, 9 collinear, 5 perpendicular, 3 vertical, 2 point on line, 1 midpoint, 1230 other
  measures "d164" distance of L1.end L2.end
  measures "d165" distance of L0.end L1.end
  measures "d168" distance of L1.end L5.end
  measures "d171" distance of L1.end L9.end
  measures "d176" distance of L0.start L32.start
  measures "d181" distance of L194.end L195.end
  measures "d189" distance of L198.end L199.end
  measures "d190" distance of L197.end L198.end
  measures "d193" distance of L197.start L201.start
  measures "d196" distance of L197.start L205.start
  measures "d201" distance of L199.end L230.end
  measures "d206" distance of L422.end L423.end
  measures "d207" distance of L426.end L427.end
  measures "d208" distance between parallel lines of L424 L395
  measures "d209" distance from line of point (154.109, 25.476) L422
  measures "d212" distance of L427.end L429.end
  measures "d215" distance of L427.end L433.end
  measures "d220" distance of L439.end L457.end
  measures "d225" distance between parallel lines of L196 L165
extrude "擠出4" cut sketch "草圖5" against normal blind 0.6 contours L0 L1 L2 L3 | L4 L5 L6 L7 | L8 L9 L10 L11 | L12 L13 L14 L15 | L16 L17 L18 L19 | L20 L21 L22 L23 | L24 L25 L26 L27 | L28 L29 L30 L31 | L32 L34 L39 L33 | L35 L37 L38 L36 | L40 L42 L43 L41 | L44 L45 L46 L47 | L48 L51 L50 L49 | L52 L55 L54 L53 | L56 L59 L58 L57 | L60 L63 L62 L61 | L64 L66 L71 L65 | L67 L69 L70 L68 | L72 L74 L75 L73 | L76 L77 L78 L79 | L80 L83 L82 L81 | L84 L87 L86 L85 | L88 L91 L90 L89 | L92 L95 L94 L93 | L96 L98 L103 L97 | L99 L101 L102 L100 | L104 L106 L107 L105 | L108 L109 L110 L111 | L112 L115 L114 L113 | L116 L119 L118 L117 | L120 L123 L122 L121 | L124 L127 L126 L125 | L128 L130 L135 L129 | L131 L133 L134 L132 | L136 L138 L139 L137 | L140 L141 L142 L143 | L144 L147 L146 L145 | L148 L151 L150 L149 | L152 L155 L154 L153 | L156 L159 L158 L157 | L160 L162 L167 L161 | L163 L165 L166 L164 | L168 L170 L171 L169 | L172 L173 L174 L175 | L176 L179 L178 L177 | L180 L183 L182 L181 | L184 L187 L186 L185 | L188 L191 L190 L189 | L197 L198 L199 L200 | L201 L203 L204 L202 | L205 L207 L208 L206 | L209 L211 L212 L210 | L213 L215 L216 L214 | L217 L219 L220 L218 | L221 L223 L224 L222 | L225 L227 L228 L226 | L229 L236 L234 L235 | L230 L231 L232 L233 | L237 L242 L243 L244 | L238 L240 L239 L241 | L245 L250 L252 L249 | L246 L247 L248 L251 | L253 L258 L260 L259 | L254 L256 L255 L257 | L261 L268 L266 L267 | L262 L263 L264 L265 | L269 L274 L275 L276 | L270 L272 L271 L273 | L277 L282 L284 L281 | L278 L279 L280 L283 | L285 L290 L292 L291 | L286 L288 L287 L289 | L293 L300 L298 L299 | L294 L295 L296 L297 | L301 L306 L307 L308 | L302 L304 L303 L305 | L309 L314 L316 L313 | L310 L311 L312 L315 | L317 L322 L324 L323 | L318 L320 L319 L321 | L325 L332 L330 L331 | L326 L327 L328 L329 | L333 L338 L339 L340 | L334 L336 L335 L337 | L341 L346 L348 L345 | L342 L343 L344 L347 | L349 L354 L356 L355 | L350 L352 L351 L353 | L357 L364 L362 L363 | L358 L359 L360 L361 | L365 L370 L371 L372 | L366 L368 L367 L369 | L373 L378 L380 L377 | L374 L375 L376 L379 | L381 L386 L388 L387 | L382 L384 L383 L385 | L389 L396 L394 L395 | L390 L391 L392 L393 | L397 L402 L403 L404 | L398 L400 L399 L401 | L405 L410 L412 L409 | L406 L407 L408 L411 | L413 L418 L420 L419 | L414 L416 L415 L417 | L425 L426 L427 L428 | L429 L430 L431 L432 | L433 L434 L435 L436 | L437 L438 L439 L440 | L441 L442 L443 L444 | L445 L446 L447 L448 | L449 L450 L451 L452 | L453 L454 L455 L456 | L457 L463 L464 L462 | L458 L461 L459 L460 | L465 L471 L472 L470 | L466 L469 L468 L467 | L473 L475 L476 L474 | L477 L479 L480 L478 | L481 L485 L483 L484 | L482 L487 L488 L486 | L489 L495 L496 L494 | L490 L493 L491 L492 | L497 L503 L504 L502 | L498 L501 L500 L499 | L505 L507 L508 L506 | L509 L511 L512 L510 | L513 L517 L515 L516 | L514 L519 L520 L518 | L521 L527 L528 L526 | L522 L525 L523 L524 | L529 L535 L536 L534 | L530 L533 L532 L531 | L537 L539 L540 L538 | L541 L543 L544 L542 | L545 L549 L547 L548 | L546 L551 L552 L550 | L553 L559 L560 L558 | L554 L557 L555 L556 | L561 L567 L568 L566 | L562 L565 L564 L563 | L569 L571 L572 L570 | L573 L575 L576 L574 | L577 L581 L579 L580 | L578 L583 L584 L582 | L585 L591 L592 L590 | L586 L589 L587 L588 | L593 L599 L600 L598 | L594 L597 L596 L595 | L601 L603 L604 L602 | L605 L607 L608 L606 | L609 L613 L611 L612 | L610 L615 L616 L614
extrude "擠出5" add sketch "草圖5" along normal blind 1.5 contours L192 L196 L193 L194 | L192 L424 L421 L422